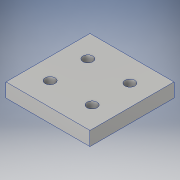
# Autodesk Inventor part: holestandard
Saved by Autodesk Inventor 2018 (Build 220112000, 112)
## iProperties
Created: 2020-10-03
Part Number: holestandard
Material: Aluminum 6061
Document SubType Name: Modeling
Designer: Lveli
Density: 2.7 g/cm^3
Appearance: Aluminum - Flat
Author: Lveli
Autodesk Inventor part; units mm, degrees
ref_plane "YZ Plane" through (0, 0, 0) normal (1, 0, 0) x (0, 1, 0)
ref_plane "XZ Plane" through (0, 0, 0) normal (0, 1, 0) x (-1, 0, 0)
ref_plane "XY Plane" through (0, 0, 0) normal (0, 0, 1) x (1, 0, 0)
sketch "Sketch1" plane through (0, 0, 0) normal (0, 1, 0) x (-1, 0, 0)
  line L0 (-19.05, 19.05) -> (19.05, 19.05)
  line L1 (19.05, 19.05) -> (19.05, -19.05)
  line L2 (19.05, -19.05) -> (-19.05, -19.05)
  line L3 (-19.05, -19.05) -> (-19.05, 19.05)
  line L4 (-19.05, 19.05) -> (19.05, -19.05) construction
  line L5 (19.05, 19.05) -> (-19.05, -19.05) construction
  point P0 (0, 0)
  dimension "d0" = 38.1
  dimension "d1" = 38.1
  constraints: 12 end point, 2 midpoint, 2 parallel, 1 horizontal, 1 perpendicular
  measures "d0" distance of L1.end L2.end
  measures "d1" distance of L0.end L1.end
extrude "Extrusion1" add sketch "Sketch1" along normal blind 6.35
sketch "Sketch2" plane through (0, 6.35, 0) normal (0, 1, 0) x (1, 0, 0)
  line L0 (-19.05, -19.05) -> (19.05, -19.05) construction
  line L1 (19.05, -19.05) -> (19.05, 19.05) construction
  line L2 (19.05, 19.05) -> (-19.05, 19.05) construction
  line L3 (-19.05, 19.05) -> (-19.05, -19.05) construction
  point P0 (0, 0)
  point P1 (-9.525, -8.5725)
  point P2 (-9.525, 8.5725)
  point P3 (9.525, -8.5725)
  point P4 (9.525, 8.5725)
  dimension "d6" = 17.145
  dimension "d9" = 19.05
  dimension "d12" = 8.5725
  dimension "d13" = 9.525
  constraints: 1 horizontal, 1 vertical, 3 other
  measures "d6" distance of point (-9.525, -8.573) point (-9.525, 8.573)
  measures "d9" distance of point (-9.525, -8.573) point (9.525, -8.573)
  measures "d12" vertical distance of point (-9.525, -8.573) point (0, 0)
  measures "d13" horizontal distance of point (-9.525, -8.573) point (0, 0)
hole "Hole1" at (-9.525, 6.35, 8.5725) at (-9.525, 6.35, -8.5725) at (9.525, 6.35, 8.5725) at (9.525, 6.35, -8.5725) direction (0, -1, 0) diameter 4.4958 end through all clearance for "Flat Head Machine Screw (82)" size "#8" standard "Ansi Unified Screw Threads"
equation "\"d12\" = 0.5 * d6"
equation "\"d13\" = 0.5 * d9"
body "Solid1"
